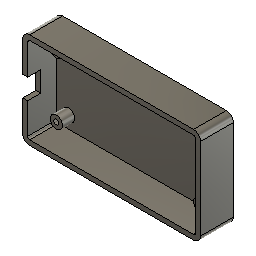
C64 KeyboardTester box v6 (Autodesk Fusion 360 design; units mm, degrees)
Autodesk Fusion 360 part; units mm, degrees
note: some values were not read from the file. Set by a fixed rule: which sketch regions a step uses.
sketch "Skizze1" plane through (0, 0, 0) normal (0, 0, 1) x (1, 0, 0) in component "Component"
  line L0 (0, 0) -> (80, 0)
  line L1 (80, 0) -> (80, 40)
  line L2 (80, 40) -> (0, 40)
  line L3 (0, 40) -> (0, 0)
  circle A0 centre (5, 5) radius 1.2
  circle A1 centre (5, 35) radius 1.2
  circle A2 centre (75, 35) radius 1.2
  circle A3 centre (75, 5) radius 1.2
  circle A4 centre (5, 35) radius 3
  circle A5 centre (5, 5) radius 3
  circle A6 centre (75, 35) radius 3
  circle A7 centre (75, 5) radius 3
  line L4 (0, 41) -> (80, 41)
  line L5 (81, 40) -> (81, 0)
  line L6 (80, -1) -> (0, -1)
  line L7 (-1, 0) -> (-1, 40)
  arc A8 (0, 41) -> (-1, 40) centre (0, 40) ccw
  line L8 (80, 0) -> (0, 0)
  line L9 (0, 0) -> (0, 40)
  line L10 (0, 40) -> (80, 40)
  line L11 (80, 40) -> (80, 0)
  arc A9 (81, 40) -> (80, 41) centre (80, 40) ccw
  arc A10 (80, -1) -> (81, 0) centre (80, 0) ccw
  arc A11 (-1, 0) -> (0, -1) centre (0, 0) ccw
  arc A12 (83.4, 40) -> (80, 43.4) centre (80, 40) ccw
  line L12 (0, 43.4) -> (80, 43.4)
  arc A13 (0, 43.4) -> (-3.4, 40) centre (0, 40) ccw
  line L13 (-3.4, 0) -> (-3.4, 40)
  arc A14 (-3.4, 0) -> (0, -3.4) centre (0, 0) ccw
  line L14 (80, -3.4) -> (0, -3.4)
  arc A15 (80, -3.4) -> (83.4, 0) centre (80, 0) ccw
  line L15 (83.4, 40) -> (83.4, 0)
  dimension "d1" = 40
  dimension "d2" = 80
  dimension "d3" = 2.4
  dimension "d4" = 2.4
  dimension "d5" = 2.4
  dimension "d6" = 2.4
  dimension "d7" = 6
  dimension "d8" = 6
  dimension "d9" = 6
  dimension "d10" = 6
  dimension "d13" = 1
  dimension "d14" = 1
  dimension "d15" = 1
  dimension "d16" = 1
  dimension "d17" = 1
  dimension "d18" = 1
  dimension "d19" = 1
  dimension "d20" = 1
  dimension "d21" = 1
  dimension "d35" = 5
  dimension "d36" = 5
  dimension "d37" = 5
  dimension "d38" = 5
  dimension "d39" = 5
  dimension "d40" = 5
  dimension "d41" = 5
  dimension "d42" = 5
  constraint horizontal L0
  constraint vertical L1
  constraint horizontal L2
  constraint vertical L3
  constraint coincident L0.start L3.end
  constraint concentric A1 A4
  constraint concentric A0 A5
  constraint concentric A2 A6
  constraint concentric A3 A7
  constraint horizontal L4
  constraint vertical L5
  constraint horizontal L6
  constraint vertical L7
  constraint tangent L4 A8
  constraint tangent L7 A8
  constraint tangent L4 A9
  constraint tangent L5 A9
  constraint tangent L5 A10
  constraint tangent L6 A10
  constraint tangent L6 A11
  constraint tangent L7 A11
  measures "d1" distance of L0.start L2.end
  measures "d2" distance of L1.end L2.end
  measures "d3" diameter of A0
  measures "d4" diameter of A1
  measures "d5" diameter of A2
  measures "d6" diameter of A3
  measures "d7" diameter of A4
  measures "d8" diameter of A5
  measures "d9" diameter of A6
  measures "d10" diameter of A7
  measures "d13" distance of L2 L4
  measures "d14" distance of L0 L6
  measures "d15" distance of L1 L5
  measures "d16" distance of L3 L7
  measures "d17" radius of A8
  measures "d19" radius of A9
  measures "d20" radius of A10
  measures "d21" radius of A11
  measures "d35" horizontal distance of A0.centre L0.start
  measures "d36" distance of A0.centre L8
  measures "d37" distance of L2 A1.centre
  measures "d38" distance of A1.centre L9
  measures "d39" distance of A2.centre L11
  measures "d40" distance of A2.centre L10
  measures "d41" distance of A3.centre L8
  measures "d42" distance of A3.centre L11
extrude "Extrusion1" add sketch "Skizze1" along normal blind 2 contours L0 L1 L2 L3 L8 L9 L10 L11 | A0 | A1 | A2 | A3 | A4 | A5 | A6 | A7 | L4 L5 L6 L7 A8 A9 A10 A11 in component "Component"
extrude "Extrusion2" add sketch "Skizze1" along normal blind 8 contours A4 | A5 | A6 | A7 in component "Component"
extrude "Extrusion5" add sketch "Skizze1" along normal blind 16 contours A12 L12 A13 L13 A14 L14 A15 L15 in component "Component"
sketch "Skizze3" plane through (-3.4, 0, 0) normal (-1, 0, 0) x (0, 0, 1) in component "Component"
  line L0 (0, 40) -> (0, 0)
  line L1 (0, 0) -> (16, 0)
  line L2 (16, 0) -> (16, 40)
  line L3 (16, 40) -> (0, 40)
  line L4 (16, 20) -> (0, 20) construction
  line L5 (21.6, 15) -> (9.6, 15)
  line L6 (9.6, 15) -> (9.6, 25)
  line L7 (9.6, 25) -> (21.6, 25)
  line L8 (21.6, 25) -> (21.6, 15)
  line L9 (21.6, 15) -> (9.6, 25) construction
  line L10 (9.6, 15) -> (21.6, 25) construction
  point P0 (15.6, 20)
  dimension "d45" = 12
  dimension "d46" = 10
  dimension "d47" = 15.6
  constraint midpoint L2 L4.start
  constraint midpoint L0 L4.end
  constraint horizontal L5
  constraint perpendicular L5 L6
  constraint parallel L5 L7
  constraint parallel L6 L8
  constraint coincident L9 P0
  constraint coincident L10 P0
  constraint coincident L4 P0
  measures "d45" distance of L6.end L7.end
  measures "d46" distance of L5.end L6.end
  measures "d47" distance of L0 P0
extrude "Extrusion6" cut sketch "Skizze3" against normal blind 5 contours L2 L5 L6 L7 in component "Component"
component "Component" placed x (1, 0, 0) y (0, 1, 0) z (0, 0, 1) at (0, 0, 0)
equation "d3 = srew_hole"
equation "d4 = srew_hole"
equation "d5 = srew_hole"
equation "d6 = srew_hole"
equation "d7 = dome_dia"
equation "d8 = dome_dia"
equation "d10 = dome_dia"
equation "d34 = -wall_thickness"
equation "srew_hole = 2.4 mm"
equation "dome_dia = 6 mm"
equation "wall_thickness = 2.4 mm"
named bodies: "C64 KeyboardTester box"
